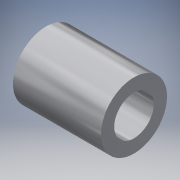
# Autodesk Inventor part: PP-I3D-0002
Saved by Autodesk Inventor 2018.3 (Build 223284000, 284)
## iProperties
Created: 2021-05-13
Part Number: PP-I3D-0002
Material: Genérico
Document SubType Name: Modeling
Designer: laguerre
Density: 8.47 g/cm^3
Appearance: Suave - Blanco
Author: laguerre
Autodesk Inventor part; units mm, degrees
ref_plane "YZ Plane" through (0, 0, 0) normal (1, 0, 0) x (0, 1, 0)
ref_plane "XZ Plane" through (0, 0, 0) normal (0, 1, 0) x (-1, 0, 0)
ref_plane "XY Plane" through (0, 0, 0) normal (0, 0, 1) x (1, 0, 0)
sketch "Boceto39" plane through (0, 0, 0) normal (0, 0, 1) x (1, 0, 0)
  circle A0 centre (0, 0) radius 2.25
  circle A1 centre (0, 0) radius 3.75
  dimension "d373" = 4.5
  dimension "d374" = 7.5
  constraints: 2 centre point, 2 coincident
  measures "d373" diameter of A0
  measures "d374" diameter of A1
extrude "Extrusión13" add sketch "Boceto39" along normal mid plane 10
